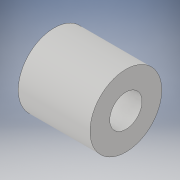
# Autodesk Inventor part: 100mm_roller
Saved by Autodesk Inventor 2019 (Build 230136000, 136)
## iProperties
Created: 2019-11-07
Part Number: 100mm_roller
Material: Generic
Document SubType Name: Modeling
Designer: luua
Density: 1 g/cm^3
Appearance: Default
Author: luua
Autodesk Inventor part; units mm, degrees
ref_plane "YZ Plane" through (0, 0, 0) normal (1, 0, 0) x (0, 1, 0)
ref_plane "XZ Plane" through (0, 0, 0) normal (0, 1, 0) x (-1, 0, 0)
ref_plane "XY Plane" through (0, 0, 0) normal (0, 0, 1) x (1, 0, 0)
sketch "Sketch1" plane through (0, 0, 0) normal (0, 0, 1) x (1, 0, 0)
  line L0 (-50, 50) -> (50, 50)
  line L1 (50, 50) -> (50, 22.5)
  line L2 (50, 22.5) -> (-50, 22.5)
  line L3 (-50, 22.5) -> (-50, 50)
  line L4 (-84.433, 0) -> (84.433, 0) construction
  point P0 (0, 0)
  point P1 (0, 0)
  point P2 (0, 22.5)
  dimension "d0" = 22.5
  dimension "d2" = 50
  dimension "d3" = 100
  constraints: 10 end point, 3 parallel, 2 horizontal, 2 midpoint, 1 coincident, 1 perpendicular, 1 vertical alignment
  measures "d0" distance between parallel lines of L4 L2
  measures "d2" distance between parallel lines of L0 L4
  measures "d3" distance of L0.start L0.end
revolve "Revolution1" add sketch "Sketch1" angle 360 about axis through (-84.433, 0, 0) along (1, 0, 0)
body "Solid1"
